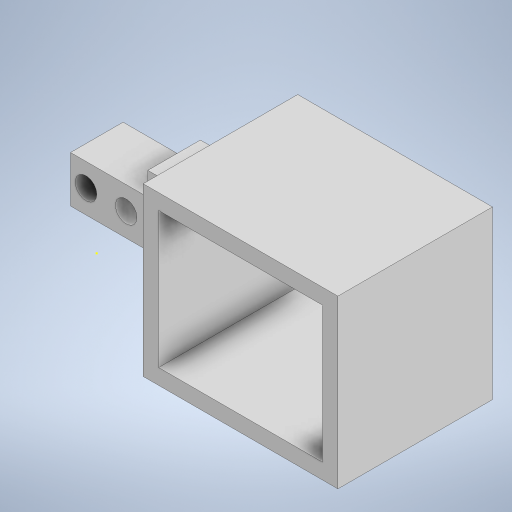
# Autodesk Inventor part: Upper_battery
Saved by Autodesk Inventor 2024 (Build 280153000, 153)
## iProperties
Created: 2024-11-10
Part Number: Upper_battery
Material: Generic
Document SubType Name: Modeling
Designer: manas
Density: 1 g/cm^3
Appearance: Default
Author: manas
Autodesk Inventor part; units mm, degrees
ref_plane "YZ Plane" through (0, 0, 0) normal (1, 0, 0) x (0, 1, 0)
ref_plane "XZ Plane" through (0, 0, 0) normal (0, 1, 0) x (-1, 0, 0)
ref_plane "XY Plane" through (0, 0, 0) normal (0, 0, 1) x (1, 0, 0)
sketch "Sketch1" plane through (0, 0, 0) normal (1, 0, 0) x (0, 1, 0)
  line L0 (-15, 8.5) -> (15, 8.5)
  line L1 (15, 8.5) -> (15, -8.5)
  line L2 (15, -8.5) -> (-15, -8.5)
  line L3 (-15, -8.5) -> (-15, 8.5)
  line L4 (-15, 8.5) -> (15, -8.5) construction
  line L5 (15, 8.5) -> (-15, -8.5) construction
  point P0 (0, 0)
  dimension "d0" = 30
  dimension "d1" = 17
  constraints: 12 end point, 2 midpoint, 2 parallel, 1 horizontal, 1 perpendicular
  measures "d0" distance of L1.end L2.end
  measures "d1" distance of L0.end L1.end
extrude "Extrusion1" add sketch "Sketch1" along normal blind 15
sketch "Sketch2" plane through (0, 0, 0) normal (-1, 0, 0) x (0, 0, 1)
  line L0 (-8.5, 7.5) -> (8.5, 7.5)
  line L1 (8.5, 7.5) -> (8.5, -7.5)
  line L2 (8.5, -7.5) -> (-8.5, -7.5)
  line L3 (-8.5, -7.5) -> (-8.5, 7.5)
  line L4 (-8.5, 7.5) -> (8.5, -7.5) construction
  line L5 (8.5, 7.5) -> (-8.5, -7.5) construction
  point P0 (0, 0)
  dimension "d4" = 17
  dimension "d5" = 15
  constraints: 12 end point, 2 midpoint, 2 parallel, 1 horizontal, 1 perpendicular
  measures "d4" distance of L1.end L2.end
  measures "d5" distance of L0.end L1.end
extrude "Extrusion2" add sketch "Sketch2" along normal blind 25
sketch "Sketch3" plane through (15, 0, 0) normal (1, 0, 0) x (0, 0, -1)
  line L0 (-25, 27) -> (25, 27)
  line L1 (25, 27) -> (25, -27)
  line L2 (25, -27) -> (-25, -27)
  line L3 (-25, -27) -> (-25, 27)
  line L4 (-25, 27) -> (25, -27) construction
  line L5 (25, 27) -> (-25, -27) construction
  point P0 (0, 0)
  dimension "d8" = 50
  dimension "d9" = 54
  constraints: 12 end point, 2 midpoint, 2 parallel, 1 horizontal, 1 perpendicular
  measures "d8" distance of L1.end L2.end
  measures "d9" distance of L0.end L1.end
extrude "Extrusion3" add sketch "Sketch3" along normal blind 5
sketch "Sketch4" plane through (20, 0, 0) normal (1, 0, 0) x (0, 0, -1)
  line L0 (-25, 27) -> (-25, -27) projected
  line L1 (-25, 27) -> (25, 27)
  line L2 (25, 27) -> (25, 22)
  line L3 (25, 22) -> (-25, 22)
  line L4 (-25, 22) -> (-25, 27)
  line L5 (-25, -27) -> (25, -27) projected
  line L6 (-25, -27) -> (25, -27)
  line L7 (25, -27) -> (25, -22)
  line L8 (25, -22) -> (-25, -22)
  line L9 (-25, -22) -> (-25, -27)
  point P0 (0, 0)
  dimension "d12" = 50
  dimension "d13" = 5
  dimension "d14" = 50
  dimension "d15" = 5
  constraints: 16 end point, 4 parallel, 2 horizontal, 2 perpendicular
  measures "d12" distance of L2.end L3.end
  measures "d13" distance of L1.end L2.end
  measures "d14" distance of L8.end L7.end
  measures "d15" distance of L7.end L6.end
extrude "Extrusion4" add sketch "Sketch4" along normal blind 58
sketch "Sketch5" plane through (20, -22, 25) normal (0, 1, 0) x (1, 0, 0)
  line L0 (0, 50) -> (58, 50) projected
  line L1 (0, 0) -> (58, 0) projected
  line L2 (58, 50) -> (53, 50)
  line L3 (53, 50) -> (53, 0)
  line L4 (53, 0) -> (58, 0)
  line L5 (58, 0) -> (58, 50)
  point P0 (-20, 25)
  dimension "d18" = 5
  constraints: 8 end point, 2 parallel, 1 horizontal, 1 perpendicular, 1 point on line
  measures "d18" distance of L4.end L3.end
extrude "Extrusion5" add sketch "Sketch5" along normal blind 45
sketch "Sketch6" plane through (15, -27, 25) normal (0, 0, 1) x (1, 0, 0)
  point P0 (-15, 27)
sketch "Sketch7" plane through (0, 7.5, 8.5) normal (0, 0, 1) x (1, 0, 0)
  line L0 (-25, 0) -> (-25, -15) projected
  line L1 (-25, -7.5) -> (-20, -7.5)
  line L2 (0, -7.5) -> (-7, -7.5)
  circle A0 centre (-7, -7.5) radius 3.5
  circle A1 centre (-20, -7.5) radius 3.5
  dimension "d21" = 5
  dimension "d22" = 7
  dimension "d23" = 7
  dimension "d24" = 7
  constraints: 4 end point, 2 centre point, 2 coincident, 2 horizontal, 1 midpoint
  measures "d21" distance of L1.start L1.end
  measures "d22" distance of L2.start L2.end
  measures "d23" diameter of A0
  measures "d24" diameter of A1
extrude "Extrusion6" cut sketch "Sketch7" against normal through all
sketch "Sketch8" plane through (0, -15, -8.5) normal (0, 0, -1) x (-1, 0, 0)
  point P0 (0, 15)
body "Solid1"
